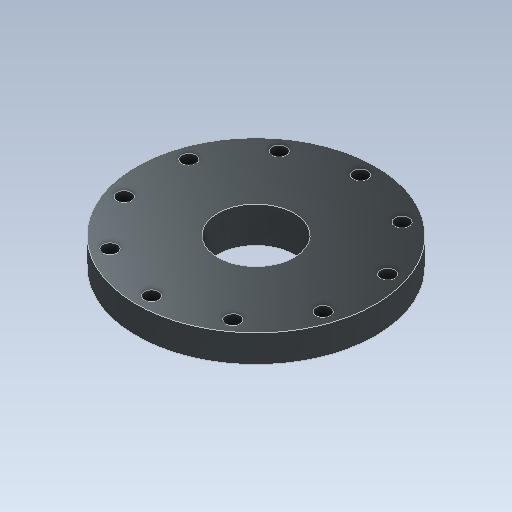
# Autodesk Inventor part: Крышка сальников_CPY
Saved by Autodesk Inventor 2021 (Build 250183000, 183)
## iProperties
Created: 2020-11-05
Part Number: Крышка сальников_CPY
Material: Чугун, серый
Document SubType Name: Modeling
Designer: Тимоха
Mass: 4950.53 g
Surface Area: 904.779 cm^2
Volume: 692.382 cm^3
Density: 7.15 g/cm^3
Appearance: Чугун серый
Author: Тимоха
Autodesk Inventor part; units mm, degrees
ref_plane "YZ Plane" through (0, 0, 0) normal (1, 0, 0) x (0, 1, 0)
ref_plane "XZ Plane" through (0, 0, 0) normal (0, 1, 0) x (-1, 0, 0)
ref_plane "XY Plane" through (0, 0, 0) normal (0, 0, 1) x (1, 0, 0)
sketch "Эскиз1" plane through (0, 0, 0) normal (0, 0, 1) x (1, 0, 0)
  line L0 (0, 0) -> (0, 18)
  line L1 (0, 18) -> (100, 18)
  line L2 (100, 18) -> (100, -5)
  line L3 (100, -5) -> (69, -5)
  line L4 (69, -5) -> (69, -12)
  line L5 (69, -12) -> (49, -12)
  line L6 (49, -12) -> (49, 1)
  line L7 (49, 1) -> (32, 1)
  line L8 (32, 1) -> (32, 18)
  line L9 (32, 1) -> (32, -12)
  line L10 (32, -12) -> (49, -12)
  dimension "d7" = 18
  dimension "d8" = 100
  dimension "d9" = 23
  dimension "d10" = 31
  dimension "d11" = 20
  dimension "d12" = 13
  dimension "d13" = 17
  dimension "d26" = 17
  constraints: 22 end point, 7 perpendicular, 3 vertical, 1 horizontal, 1 point on line
  measures "d7" distance of L0.start L0.end
  measures "d8" distance of L0.end L1.end
  measures "d9" distance of L1.end L2.end
  measures "d10" distance of L2.end L3.end
  measures "d11" distance of L4.end L5.end
  measures "d12" distance of L5.end L6.end
  measures "d13" distance of L6.end L7.end
  measures "d26" distance of L7.end L8.end
revolve "Вращение1" add sketch "Эскиз1" angle 360 about axis through (0, 0, 0) along (0, 1, 0)
sketch "Эскиз2" plane through (0, 18, 0) normal (0, 1, 0) x (1, 0, 0)
  circle A0 centre (0, 0) radius 100 projected
  circle A1 centre (0, 0) radius 100 projected
  line L0 (0, 100) -> (0, 87.5)
  dimension "d15" = 12.5
  constraints: 2 end point, 1 vertical, 1 vertical alignment, 1 other
  measures "d15" distance of L0.start L0.end
hole "Отверстие1" at (0, 18, -87.5) direction (0, -1, 0) diameter 12 end through all
pattern_circular "Круговой массив2" count 10 over 360 about axis through (0, 6.5, 0) along (0, -1, 0) of "Отверстие1"
